Autodesk Inventor part; units mm, degrees
note: some values were not read from the file. Chosen so that the rebuilt part matches the saved one: direction of "Hole2".
(part 3 of 20)
  line L329 (-10082.582375, -10027.370137) -> (-10083.030705, -10031.210292)
  ellipse E243 centre (-10082.779407, -10029.059983) end of major axis (-10083.069525, -10031.543092) minor radius 0.000126 (-10083.029846, -10031.202932) -> (-10083.069521, -10031.543049) ccw
  line L330 (-10085.513815, -10030.920174) -> (-10085.181506, -10028.073798)
  ellipse E244 centre (-10085.262516, -10028.769865) end of major axis (-10085.552634, -10031.252974) minor radius 0.000126 (-10085.513815, -10030.920174) -> (-10085.552634, -10031.252974) ccw
  line L331 (-10083.069525, -10031.543092) -> (-10085.552634, -10031.252974)
  ellipse E245 centre (-10082.117991, -10023.398136) end of major axis (-10083.104393, -10031.840708) minor radius 0.000429 (-10083.054997, -10031.419086) -> (-10082.967028, -10030.666888) ccw
  line L332 (-10084.568877, -10027.13817) -> (-10084.684884, -10028.131821)
  ellipse E246 centre (-10082.643707, -10010.297398) end of major axis (-10082.614695, -10010.545709) minor radius 0.000013
  ellipse E247 centre (-10082.518842, -10011.365844) end of major axis (-10082.588111, -10010.772977) minor radius 0.00003 (-10082.582158, -10010.823819) -> (-10082.582182, -10010.823822) ccw
  ellipse E248 centre (-10082.117991, -10014.795845) end of major axis (-10083.104393, -10006.353274) minor radius 0.000429 (-10082.967028, -10007.527094) -> (-10083.054997, -10006.774896) ccw
  ellipse E249 centre (-10082.779407, -10009.133999) end of major axis (-10083.069525, -10006.650889) minor radius 0.000126 (-10083.054997, -10006.774896) -> (-10083.030705, -10006.983689) ccw
  line L333 (-10083.030705, -10006.983689) -> (-10082.582375, -10010.823844)
  line L334 (-10085.181506, -10010.120184) -> (-10085.513815, -10007.273807)
  ellipse E250 centre (-10085.262516, -10009.424117) end of major axis (-10085.552634, -10006.941007) minor radius 0.000126 (-10085.552634, -10006.941007) -> (-10085.513815, -10007.273807) ccw
  line L335 (-10085.552634, -10006.941007) -> (-10083.069525, -10006.650889)
  ellipse E251 centre (-10082.926301, -10007.876835) end of major axis (-10082.833946, -10008.667304) minor radius 0.000039 (-10082.96711, -10007.527248) -> (-10082.967167, -10007.527356) ccw
  line L336 (-10084.684884, -10010.06216) -> (-10084.568877, -10011.055811)
  line L337 (-10088.375684, -10026.030053) -> (-10088.470056, -10027.025887)
  line L338 (-10089.238176, -10029.831508) -> (-10088.967825, -10026.978705)
  ellipse E252 centre (-10089.033868, -10027.676195) end of major axis (-10089.269776, -10030.16504) minor radius 0.000028 (-10089.238176, -10029.831508) -> (-10089.269776, -10030.16504) ccw
  line L339 (-10087.361677, -10030.345901) -> (-10089.269776, -10030.16504)
  line L340 (-10088.55652, -10015.008914) -> (-10088.570909, -10015.096991)
  line L341 (-10088.570909, -10023.096991) -> (-10088.55652, -10023.185067)
  line L342 (-10088.777126, -10024.881551) -> (-10088.905304, -10024.096991)
  line L343 (-10088.905304, -10014.096991) -> (-10088.777126, -10013.312431)
  line L344 (-10088.470056, -10011.168095) -> (-10088.375684, -10012.163929)
  line L345 (-10088.967825, -10011.215277) -> (-10089.238176, -10008.362473)
  ellipse E253 centre (-10089.033868, -10010.517786) end of major axis (-10089.269776, -10008.028942) minor radius 0.000028 (-10089.269776, -10008.028942) -> (-10089.238179, -10008.362444) ccw
  line L346 (-10089.269776, -10008.028942) -> (-10087.361677, -10007.84808)
  spline S0 degree 3 poles (-10089.355394, -10025.372994) (-10089.375203, -10025.328104) (-10089.41441, -10025.239254) (-10089.470581, -10025.106444) (-10089.524077, -10024.975666) (-10089.590992, -10024.805344) (-10089.66863, -10024.596725) (-10089.723709, -10024.42915) (-10089.750761, -10024.346845) knots 0 0 0 0 0.13378969 0.26480564 0.39318317 0.51905417 0.76378306 1 1 1 1
  line L347 (-10088.828929, -10025.428076) -> (-10089.355394, -10025.372994)
  spline S1 degree 3 poles (-10089.713059, -10026.50077) (-10089.711978, -10026.51419) (-10089.709847, -10026.540646) (-10089.707768, -10026.579767) (-10089.706628, -10026.617583) (-10089.706543, -10026.653893) (-10089.707549, -10026.688508) (-10089.709676, -10026.721288) (-10089.712863, -10026.752152) (-10089.717058, -10026.781056) (-10089.722211, -10026.807959) (-10089.728269, -10026.832818) (-10089.735181, -10026.855595) (-10089.742902, -10026.876266) (-10089.751482, -10026.894991) (-10089.761038, -10026.911918) (-10089.771484, -10026.927357) (-10089.779493, -10026.936504) (-10089.783423, -10026.940992) knots 0 0 0 0 0.08847523 0.17442408 0.25743028 0.33708941 0.41301484 0.48496567 0.5529194 0.61687848 0.67685349 0.73286663 0.78495643 0.83318442 0.87777974 0.92016243 0.96082909 1 1 1 1
  ellipse E254 centre (-10089.027378, -10022.2409) end of major axis (-10089.595637, -10027.672254) minor radius 0.000387 (-10089.355394, -10025.372995) -> (-10089.595637, -10027.672254) ccw
  line L348 (-10089.849985, -10027.358464) -> (-10089.595637, -10027.672254)
  line L349 (-10089.039069, -10027.730485) -> (-10089.595637, -10027.672254)
  spline S2 degree 3 poles (-10089.491941, -10022.246911) (-10089.516181, -10022.204326) (-10089.564161, -10022.120035) (-10089.633469, -10021.993791) (-10089.69992, -10021.869289) (-10089.78374, -10021.706851) (-10089.882131, -10021.507435) (-10089.953949, -10021.346516) (-10089.989225, -10021.267475) knots 0 0 0 0 0.13376268 0.26475964 0.39312605 0.51899363 0.76373828 1 1 1 1
  line L350 (-10089.310215, -10022.246911) -> (-10089.491941, -10022.246911)
  line L351 (-10089.491941, -10015.94707) -> (-10089.310215, -10015.94707)
  spline S3 degree 3 poles (-10089.989225, -10016.926507) (-10089.953949, -10016.847466) (-10089.882131, -10016.686546) (-10089.78374, -10016.487131) (-10089.69992, -10016.324692) (-10089.633469, -10016.200191) (-10089.564161, -10016.073947) (-10089.516181, -10015.989656) (-10089.491941, -10015.94707) knots 0 0 0 0 0.23626172 0.48100637 0.60687395 0.73524036 0.86623732 1 1 1 1
  line L352 (-10089.989225, -10021.267475) -> (-10089.989225, -10016.926507)
  ellipse E255 centre (-10089.524961, -10019.096991) end of major axis (-10089.524961, -10024.057991) minor radius 0.5163 (-10089.959804, -10016.422408) -> (-10089.989225, -10016.926507) ccw
  ellipse E256 centre (-10089.524961, -10019.096991) end of major axis (-10089.524961, -10024.057991) minor radius 0.5163 (-10089.989225, -10021.267475) -> (-10089.959804, -10021.771573) ccw
  ellipse E257 centre (-10089.027676, -10019.096991) end of major axis (-10089.027676, -10013.635991) minor radius 0.568336 (-10089.165773, -10013.799655) -> (-10089.491941, -10015.94707) ccw
  ellipse E258 centre (-10089.027676, -10019.096991) end of major axis (-10089.027676, -10024.557991) minor radius 0.568336 (-10089.491941, -10022.246911) -> (-10089.165773, -10024.394327) ccw
  line L353 (-10089.355394, -10012.820988) -> (-10088.828929, -10012.765906)
  spline S4 degree 3 poles (-10089.750761, -10013.847136) (-10089.723709, -10013.764832) (-10089.66863, -10013.597256) (-10089.590992, -10013.388638) (-10089.524077, -10013.218316) (-10089.470581, -10013.087538) (-10089.41441, -10012.954727) (-10089.375203, -10012.865878) (-10089.355394, -10012.820988) knots 0 0 0 0 0.23621694 0.48094583 0.60681683 0.73519436 0.86621031 1 1 1 1
  spline S5 degree 3 poles (-10089.783618, -10011.253438) (-10089.779613, -10011.258107) (-10089.771405, -10011.267675) (-10089.76069, -10011.283901) (-10089.750805, -10011.301818) (-10089.74191, -10011.321545) (-10089.733975, -10011.343026) (-10089.727027, -10011.366257) (-10089.721076, -10011.391219) (-10089.716138, -10011.417899) (-10089.712225, -10011.446299) (-10089.709353, -10011.476466) (-10089.707507, -10011.508436) (-10089.70667, -10011.542209) (-10089.706829, -10011.57773) (-10089.707995, -10011.614936) (-10089.710092, -10011.653771) (-10089.712241, -10011.68016) (-10089.713337, -10011.693625) knots 0 0 0 0 0.04039145 0.08278851 0.12750015 0.17478558 0.22486002 0.27790108 0.33405492 0.39344169 0.45616024 0.52241148 0.59256068 0.66658365 0.74441779 0.82598879 0.91121312 1 1 1 1
  ellipse E259 centre (-10089.027378, -10015.953082) end of major axis (-10089.595637, -10010.521728) minor radius 0.000387 (-10089.595637, -10010.521728) -> (-10089.355394, -10012.820988) ccw
  line L354 (-10089.849985, -10010.835518) -> (-10089.595637, -10010.521728)
  line L355 (-10089.039069, -10010.463496) -> (-10089.595637, -10010.521728)
  spline S6 degree 3 poles (-10091.282091, -10024.900964) (-10091.302336, -10024.856269) (-10091.342408, -10024.767806) (-10091.39987, -10024.635549) (-10091.454637, -10024.505299) (-10091.523209, -10024.335637) (-10091.602875, -10024.127785) (-10091.659584, -10023.960754) (-10091.687437, -10023.878716) knots 0 0 0 0 0.13378969 0.26480564 0.39318317 0.51905417 0.76378306 1 1 1 1
  line L356 (-10089.484899, -10025.071313) -> (-10091.282091, -10024.900964)
  line L357 (-10091.687437, -10023.878716) -> (-10091.612013, -10023.082983)
  ellipse E260 centre (-10091.482604, -10021.718237) end of major axis (-10091.950739, -10026.6571) minor radius 0.000055 (-10091.93466, -10026.487305) -> (-10091.950739, -10026.6571) ccw
  ellipse E261 centre (-10091.482604, -10021.718237) end of major axis (-10091.950739, -10026.6571) minor radius 0.000055 (-10091.687437, -10023.878716) -> (-10091.814007, -10025.21415) ccw
  spline S7 degree 3 poles (-10091.814007, -10025.21415) (-10091.798163, -10025.265719) (-10091.767127, -10025.36673) (-10091.726257, -10025.516101) (-10091.691249, -10025.659093) (-10091.662778, -10025.794864) (-10091.640895, -10025.9237) (-10091.626418, -10026.045317) (-10091.620703, -10026.141851) (-10091.621057, -10026.213481) (-10091.623808, -10026.261718) (-10091.628873, -10026.305789) (-10091.636083, -10026.34554) (-10091.645286, -10026.380851) (-10091.659407, -10026.420321) (-10091.682241, -10026.461662) (-10091.720137, -10026.498843) (-10091.767469, -10026.519811) (-10091.821022, -10026.522371) (-10091.877958, -10026.511191) (-10091.915164, -10026.495517) (-10091.934659, -10026.487304) knots 0 0 0 0 0.10413454 0.20397599 0.29888876 0.38827472 0.47171081 0.55106733 0.62459732 0.65820388 0.68929134 0.71781594 0.74378428 0.76721832 0.78816557 0.82463321 0.85738378 0.88888098 0.92222056 0.95924484 1 1 1 1
  ellipse E262 centre (-10090.984835, -10021.765419) end of major axis (-10091.500152, -10027.202051) minor radius 0.000061 (-10091.282095, -10024.901006) -> (-10091.500152, -10027.202051) ccw
  line L358 (-10091.950739, -10026.6571) -> (-10091.500152, -10027.202051)
  ellipse E263 centre (-10091.808499, -10025.15622) end of major axis (-10091.665888, -10023.651664) minor radius 0.000017 (-10091.934703, -10026.487762) -> (-10091.821814, -10025.296875) ccw
  line L359 (-10089.849985, -10027.358464) -> (-10091.500152, -10027.202051)
  spline S8 degree 3 poles (-10091.405595, -10022.246911) (-10091.42986, -10022.204326) (-10091.477886, -10022.120036) (-10091.547262, -10021.993791) (-10091.613777, -10021.86929) (-10091.697679, -10021.706852) (-10091.796165, -10021.507438) (-10091.868055, -10021.346516) (-10091.903366, -10021.267475) knots 0 0 0 0 0.13376751 0.26476787 0.39313627 0.51900446 0.76374629 1 1 1 1
  line L360 (-10089.691497, -10022.246911) -> (-10091.405595, -10022.246911)
  line L361 (-10091.405595, -10015.94707) -> (-10089.691497, -10015.94707)
  spline S9 degree 3 poles (-10091.903366, -10016.926507) (-10091.868055, -10016.847466) (-10091.796165, -10016.686543) (-10091.697679, -10016.487129) (-10091.613777, -10016.324692) (-10091.547262, -10016.20019) (-10091.477886, -10016.073946) (-10091.42986, -10015.989656) (-10091.405595, -10015.94707) knots 0 0 0 0 0.23625371 0.48099554 0.60686373 0.73523213 0.86623249 1 1 1 1
  line L362 (-10091.903366, -10021.267475) -> (-10091.903366, -10016.926507)
  ellipse E264 centre (-10091.482582, -10019.096991) end of major axis (-10091.482582, -10024.057991) minor radius 0.467946 (-10091.813104, -10015.585157) -> (-10091.903366, -10016.926507) ccw
  ellipse E265 centre (-10091.482582, -10019.096991) end of major axis (-10091.482582, -10024.057991) minor radius 0.467946 (-10091.903366, -10021.267475) -> (-10091.813104, -10022.608825) ccw
  spline S10 degree 3 poles (-10091.813104, -10022.608825) (-10091.794916, -10022.648919) (-10091.759087, -10022.727902) (-10091.708202, -10022.845276) (-10091.6607, -10022.959182) (-10091.616959, -10023.069176) (-10091.577206, -10023.174758) (-10091.541408, -10023.276157) (-10091.509741, -10023.373699) (-10091.482497, -10023.466914) (-10091.460403, -10023.553917) (-10091.444493, -10023.632581) (-10091.434982, -10023.701386) (-10091.431489, -10023.75949) (-10091.433695, -10023.80769) (-10091.442096, -10023.846389) (-10091.455729, -10023.877879) (-10091.471318, -10023.891426) (-10091.478563, -10023.897722) knots 0 0 0 0 0.09648314 0.19006443 0.28034292 0.36693478 0.44946267 0.527566 0.60257164 0.67417927 0.74035842 0.79922956 0.84998037 0.89243012 0.92670891 0.95522625 0.97919149 1 1 1 1
  spline S11 degree 3 poles (-10091.478569, -10014.296272) (-10091.471499, -10014.302418) (-10091.456208, -10014.315713) (-10091.442744, -10014.346899) (-10091.434361, -10014.385571) (-10091.431755, -10014.433144) (-10091.434624, -10014.489116) (-10091.443205, -10014.553706) (-10091.457617, -10014.626897) (-10091.477678, -10014.708609) (-10091.503233, -10014.798357) (-10091.534062, -10014.895415) (-10091.569942, -10014.999051) (-10091.610624, -10015.108521) (-10091.655873, -10015.222921) (-10091.722241, -10015.383074) (-10091.776464, -10015.503669) (-10091.813104, -10015.585157) knots 0 0 0 0 0.02031374 0.04393674 0.07255557 0.10706143 0.14790384 0.19530387 0.24973648 0.31134419 0.37967367 0.4542385 0.53453299 0.62003981 0.71019877 0.8041769 1 1 1 1
  ellipse E266 centre (-10090.984812, -10019.096991) end of major axis (-10090.984812, -10013.635991) minor radius 0.515109 (-10091.154807, -10013.941946) -> (-10091.405595, -10015.94707) ccw
  ellipse E267 centre (-10090.984812, -10019.096991) end of major axis (-10090.984812, -10024.557991) minor radius 0.515109 (-10091.405595, -10022.246911) -> (-10091.154807, -10024.252035) ccw
  line L363 (-10091.282091, -10013.293017) -> (-10089.484899, -10013.122668)
  spline S12 degree 3 poles (-10091.687437, -10014.315265) (-10091.659584, -10014.233228) (-10091.602875, -10014.066197) (-10091.523209, -10013.858345) (-10091.454637, -10013.688683) (-10091.39987, -10013.558433) (-10091.342408, -10013.426176) (-10091.302336, -10013.337712) (-10091.282091, -10013.293017) knots 0 0 0 0 0.23621694 0.48094583 0.60681683 0.73519436 0.86621031 1 1 1 1
  line L364 (-10091.612013, -10015.110999) -> (-10091.687437, -10014.315265)
  ellipse E268 centre (-10091.482604, -10016.475744) end of major axis (-10091.014468, -10021.414608) minor radius 0.000055 (-10091.814145, -10012.978375) -> (-10091.687613, -10014.313411) ccw
  ellipse E269 centre (-10091.482604, -10016.475744) end of major axis (-10091.950739, -10011.536881) minor radius 0.000055 (-10091.950739, -10011.536881) -> (-10091.934659, -10011.706679) ccw
  spline S13 degree 3 poles (-10091.934659, -10011.706678) (-10091.914651, -10011.69823) (-10091.877086, -10011.68237) (-10091.820071, -10011.671463) (-10091.767544, -10011.674319) (-10091.721092, -10011.694698) (-10091.683481, -10011.731672) (-10091.654843, -10011.783177) (-10091.634672, -10011.848527) (-10091.622919, -10011.927815) (-10091.619845, -10012.021105) (-10091.624909, -10012.128035) (-10091.638005, -10012.247654) (-10091.658962, -10012.378555) (-10091.687598, -10012.519238) (-10091.723631, -10012.667871) (-10091.765738, -10012.822577) (-10091.79775, -10012.92687) (-10091.814007, -10012.979832) knots 0 0 0 0 0.04184874 0.07857029 0.11114659 0.14190435 0.17426777 0.21118388 0.25459927 0.30565856 0.36551927 0.43456112 0.51220716 0.59775966 0.69045627 0.7893544 0.8930296 1 1 1 1
  ellipse E270 centre (-10090.984835, -10016.428563) end of major axis (-10091.500152, -10010.991931) minor radius 0.000061 (-10091.500152, -10010.991931) -> (-10091.282091, -10013.293017) ccw
  line L365 (-10091.950739, -10011.536881) -> (-10091.500152, -10010.991931)
  line L366 (-10089.849985, -10010.835518) -> (-10091.500152, -10010.991931)
  ellipse E271 centre (-10092.011091, -10021.928727) end of major axis (-10092.418478, -10025.822473) minor radius 0.000278 (-10092.049003, -10022.288426) -> (-10092.181257, -10023.552725) ccw
  ellipse E272 centre (-10092.214166, -10023.867654) end of major axis (-10092.193354, -10023.66874) minor radius 0.000014 (-10092.202773, -10023.758879) -> (-10092.193354, -10023.66874) ccw
  line L367 (-10092.193376, -10023.668676) -> (-10092.193354, -10023.66874)
  ellipse E273 centre (-10092.172564, -10023.469762) end of major axis (-10092.193376, -10023.668676) minor radius 0.000014 (-10092.181257, -10023.552725) -> (-10092.193376, -10023.668676) ccw
  ellipse E274 centre (-10092.011091, -10021.928727) end of major axis (-10092.361246, -10025.275459) minor radius 0.000239 (-10092.202773, -10023.758879) -> (-10092.361246, -10025.275459) ccw
  line L368 (-10092.361246, -10025.275459) -> (-10091.825101, -10025.331553)
  ellipse E275 centre (-10107.725317, -10020.284613) end of major axis (-10107.960488, -10022.532344) minor radius 0.00016 (-10107.931882, -10022.258193) -> (-10107.960488, -10022.532344) ccw
  line L369 (-10107.960488, -10022.532344) -> (-10106.013379, -10022.828708)
  line L370 (-10091.903366, -10017.346991) -> (-10092.362753, -10017.346991)
  ellipse E276 centre (-10092.362753, -10017.546991) end of major axis (-10092.362753, -10017.346991) minor radius 0.020814 (-10092.362753, -10017.346991) -> (-10092.381669, -10017.463545) ccw
  ellipse E277 centre (-10092.011385, -10019.096991) end of major axis (-10092.011385, -10023.011991) minor radius 0.407441 (-10092.381669, -10017.463545) -> (-10092.381669, -10020.730436) ccw
  ellipse E278 centre (-10092.321979, -10017.146991) end of major axis (-10092.321979, -10017.346991) minor radius 0.020814 (-10092.321979, -10017.346991) -> (-10092.304554, -10017.256388) ccw
  ellipse E279 centre (-10092.321979, -10021.046991) end of major axis (-10092.321979, -10020.846991) minor radius 0.020814 (-10092.304554, -10020.937594) -> (-10092.321979, -10020.846991) ccw
  ellipse E280 centre (-10092.362753, -10020.646991) end of major axis (-10092.362753, -10020.846991) minor radius 0.020814 (-10092.381669, -10020.730436) -> (-10092.362753, -10020.846991) ccw
  line L371 (-10092.362753, -10020.846991) -> (-10091.903366, -10020.846991)
  ellipse E281 centre (-10092.011385, -10019.096991) end of major axis (-10092.011385, -10015.731991) minor radius 0.350202 (-10092.063275, -10015.769135) -> (-10092.304554, -10017.256388) ccw
  ellipse E282 centre (-10092.011385, -10019.096991) end of major axis (-10092.011385, -10022.461991) minor radius 0.350202 (-10092.304554, -10020.937594) -> (-10092.063275, -10022.424847) ccw
  ellipse E283 centre (-10107.725588, -10019.096991) end of major axis (-10107.725588, -10016.836991) minor radius 0.235202 (-10107.934511, -10018.058913) -> (-10107.934511, -10020.135069) ccw
  ellipse E284 centre (-10092.172564, -10014.724219) end of major axis (-10092.193376, -10014.525305) minor radius 0.000014 (-10092.193376, -10014.525305) -> (-10092.181257, -10014.641257) ccw
  ellipse E285 centre (-10092.011091, -10016.265255) end of major axis (-10091.603705, -10020.159001) minor radius 0.000278 (-10092.181259, -10014.641244) -> (-10092.049005, -10015.905542) ccw
  line L372 (-10092.193354, -10014.525241) -> (-10092.193376, -10014.525305)
  ellipse E286 centre (-10092.214166, -10014.326327) end of major axis (-10092.193354, -10014.525241) minor radius 0.000014 (-10092.193354, -10014.525241) -> (-10092.202773, -10014.435103) ccw
  ellipse E287 centre (-10092.011091, -10016.265255) end of major axis (-10092.361246, -10012.918523) minor radius 0.000239 (-10092.361246, -10012.918523) -> (-10092.202773, -10014.435105) ccw
  line L373 (-10092.361246, -10012.918523) -> (-10091.825101, -10012.862428)
  ellipse E288 centre (-10107.725317, -10017.909368) end of major axis (-10107.960488, -10015.661637) minor radius 0.00016 (-10107.960488, -10015.661637) -> (-10107.931882, -10015.935788) ccw
  line L374 (-10107.960488, -10015.661637) -> (-10106.013379, -10015.365274)
  ellipse E289 centre (-10105.757191, -10020.636212) end of major axis (-10106.019458, -10022.880943) minor radius 0.000114 (-10105.930965, -10022.122802) -> (-10106.019458, -10022.880943) ccw
  line L375 (-10106.019458, -10022.880943) -> (-10094.287038, -10024.811778)
  line L376 (-10093.990126, -10024.860641) -> (-10092.346221, -10025.131183)
  ellipse E290 centre (-10090.064389, -10019.096991) end of major axis (-10090.064389, -10023.011991) minor radius 0.45382 (-10090.510503, -10018.378625) -> (-10090.512583, -10018.482465) ccw
  ellipse E291 centre (-10090.064389, -10019.096991) end of major axis (-10090.064389, -10023.011991) minor radius 0.45382 (-10090.516487, -10018.756319) -> (-10090.515885, -10019.492622) ccw
  ellipse E292 centre (-10090.064389, -10019.096991) end of major axis (-10090.064389, -10023.011991) minor radius 0.45382 (-10090.512583, -10019.711517) -> (-10090.510503, -10019.815357) ccw
  ellipse E293 centre (-10105.757877, -10019.096991) end of major axis (-10105.757877, -10016.836991) minor radius 0.261975 (-10105.929305, -10017.38803) -> (-10105.929305, -10020.805951) ccw
  ellipse E294 centre (-10105.757191, -10017.55777) end of major axis (-10106.019458, -10015.313039) minor radius 0.000114 (-10106.019458, -10015.313039) -> (-10105.930965, -10016.07118) ccw
  line L377 (-10106.019458, -10015.313039) -> (-10094.287038, -10013.382204)
  line L378 (-10093.990126, -10013.33334) -> (-10092.346221, -10013.062799)
  ellipse E295 centre (-10110.685615, -10019.898058) end of major axis (-10110.66627, -10019.693973) minor radius 0.000002 (-10110.66627, -10019.693973) -> (-10110.689578, -10019.939846) ccw
  ellipse E296 centre (-10110.251606, -10019.939196) end of major axis (-10110.368144, -10021.168686) minor radius 0.000014 (-10110.284172, -10020.282632) -> (-10110.368144, -10021.168686) ccw
  line L379 (-10110.368144, -10021.168686) -> (-10109.817506, -10021.220878)
  arc A0 (-10110.696073, -10020.26555) -> (-10110.368144, -10021.168686) centre (-10108.775104, -10020.079148) ccw
  arc A1 (-10110.641595, -10019.588148) -> (-10110.66627, -10019.693973) centre (-10108.775104, -10020.079148) ccw
  ellipse E297 centre (-10093.971448, -10021.482329) end of major axis (-10094.34088, -10025.37986) minor radius 0.000044 (-10094.031971, -10022.120387) -> (-10094.125601, -10023.108231) ccw
  ellipse E298 centre (-10092.975911, -10021.576692) end of major axis (-10093.345342, -10025.474223) minor radius 0.000044 (-10092.99969, -10021.827109) -> (-10093.130063, -10023.202594) ccw
  line L380 (-10094.136599, -10023.224279) -> (-10094.136597, -10023.224307)
  line L381 (-10093.141061, -10023.318642) -> (-10093.141059, -10023.31867)
  ellipse E299 centre (-10093.971448, -10021.482329) end of major axis (-10094.28898, -10024.832314) minor radius 0.000037 (-10094.145146, -10023.314518) -> (-10094.28898, -10024.832314) ccw
  ellipse E300 centre (-10092.975911, -10021.576692) end of major axis (-10093.293443, -10024.926677) minor radius 0.000037 (-10093.149608, -10023.40888) -> (-10093.270588, -10024.685411) ccw
  line L382 (-10094.28898, -10024.832314) -> (-10093.990122, -10024.860642)
  ellipse E301 centre (-10109.700946, -10019.991391) end of major axis (-10109.914207, -10022.241307) minor radius 0.000025 (-10109.803801, -10021.076282) -> (-10109.914207, -10022.241307) ccw
  line L383 (-10109.914207, -10022.241307) -> (-10107.959153, -10022.519419)
  ellipse E302 centre (-10110.251653, -10019.096991) end of major axis (-10110.251653, -10017.861991) minor radius 0.116491 (-10110.284248, -10017.911323) -> (-10110.284248, -10020.282659) ccw
  arc A2 (-10110.694309, -10019.301148) -> (-10110.436834, -10020.078653) centre (-10108.775145, -10019.096991) ccw
  arc A3 (-10110.436834, -10018.115328) -> (-10110.694309, -10018.892833) centre (-10108.775145, -10019.096991) ccw
  ellipse E303 centre (-10093.294355, -10017.546991) end of major axis (-10093.294355, -10017.346991) minor radius 0.018865 (-10093.294355, -10017.346991) -> (-10093.311499, -10017.463545) ccw
  line L384 (-10093.294355, -10017.346991) -> (-10094.289896, -10017.346991)
  ellipse E304 centre (-10094.289896, -10017.546991) end of major axis (-10094.289896, -10017.346991) minor radius 0.018865 (-10094.289896, -10017.346991) -> (-10094.307041, -10017.463545) ccw
  ellipse E305 centre (-10093.971436, -10019.096991) end of major axis (-10093.971436, -10023.011991) minor radius 0.369282 (-10094.307041, -10017.463545) -> (-10094.307041, -10020.730436) ccw
  ellipse E306 centre (-10092.975894, -10019.096991) end of major axis (-10092.975894, -10023.011991) minor radius 0.369282 (-10093.311499, -10017.463545) -> (-10093.311499, -10020.730436) ccw
  ellipse E307 centre (-10094.252941, -10017.146991) end of major axis (-10094.252941, -10017.346991) minor radius 0.018865 (-10094.252941, -10017.346991) -> (-10094.237148, -10017.256388) ccw
  ellipse E308 centre (-10094.252941, -10021.046991) end of major axis (-10094.252941, -10020.846991) minor radius 0.018865 (-10094.237148, -10020.937594) -> (-10094.252941, -10020.846991) ccw
  ellipse E309 centre (-10094.289896, -10020.646991) end of major axis (-10094.289896, -10020.846991) minor radius 0.018865 (-10094.307041, -10020.730436) -> (-10094.289896, -10020.846991) ccw
  ellipse E310 centre (-10093.294355, -10020.646991) end of major axis (-10093.294355, -10020.846991) minor radius 0.018865 (-10093.311499, -10020.730436) -> (-10093.294355, -10020.846991) ccw
  line L385 (-10094.289896, -10020.846991) -> (-10093.294355, -10020.846991)
  ellipse E311 centre (-10093.257399, -10017.146991) end of major axis (-10093.257399, -10017.346991) minor radius 0.018865 (-10093.257399, -10017.346991) -> (-10093.241607, -10017.256388) ccw
  line L386 (-10093.257399, -10017.346991) -> (-10093.294355, -10017.346991)
  ellipse E312 centre (-10093.257399, -10021.046991) end of major axis (-10093.257399, -10020.846991) minor radius 0.018865 (-10093.241607, -10020.937594) -> (-10093.257399, -10020.846991) ccw
  line L387 (-10093.294355, -10020.846991) -> (-10093.257399, -10020.846991)
  ellipse E313 centre (-10093.971436, -10019.096991) end of major axis (-10093.971436, -10015.731991) minor radius 0.317404 (-10094.053503, -10015.846416) -> (-10094.237148, -10017.256388) ccw
  ellipse E314 centre (-10093.971436, -10019.096991) end of major axis (-10093.971436, -10022.461991) minor radius 0.317404 (-10094.237148, -10020.937594) -> (-10094.053503, -10022.347566) ccw
  ellipse E315 centre (-10092.975894, -10019.096991) end of major axis (-10092.975894, -10022.461991) minor radius 0.317404 (-10093.050842, -10022.366837) -> (-10093.015075, -10022.436255) ccw
  ellipse E316 centre (-10092.975894, -10019.096991) end of major axis (-10092.975894, -10015.731991) minor radius 0.317404 (-10093.241607, -10020.937594) -> (-10093.107762, -10022.157837) ccw
  ellipse E317 centre (-10092.975894, -10019.096991) end of major axis (-10092.975894, -10015.731991) minor radius 0.317404 (-10093.107762, -10016.036144) -> (-10093.241607, -10017.256388) ccw
  ellipse E318 centre (-10092.975894, -10019.096991) end of major axis (-10092.975894, -10015.731991) minor radius 0.317404 (-10093.015075, -10015.757727) -> (-10093.050842, -10015.827145) ccw
  ellipse E319 centre (-10109.700991, -10019.096991) end of major axis (-10109.700991, -10016.836991) minor radius 0.213175 (-10109.803832, -10017.117374) -> (-10109.803832, -10021.076608) ccw
  ellipse E320 centre (-10110.685615, -10018.295923) end of major axis (-10110.66627, -10018.500009) minor radius 0.000002 (-10110.689578, -10018.254136) -> (-10110.66627, -10018.500009) ccw
  ellipse E321 centre (-10110.251606, -10018.254785) end of major axis (-10110.368144, -10017.025296) minor radius 0.000014 (-10110.368144, -10017.025296) -> (-10110.284172, -10017.91135) ccw
  line L388 (-10110.368144, -10017.025296) -> (-10109.817506, -10016.973103)
  arc A4 (-10110.66627, -10018.500009) -> (-10110.641595, -10018.605833) centre (-10108.775104, -10018.114833) ccw
  arc A5 (-10110.368144, -10017.025296) -> (-10110.696073, -10017.928432) centre (-10108.775104, -10018.114833) ccw
  ellipse E322 centre (-10093.971448, -10016.711652) end of major axis (-10093.602017, -10020.609183) minor radius 0.000044 (-10094.12565, -10015.085235) -> (-10094.032024, -10016.073035) ccw
  ellipse E323 centre (-10092.975911, -10016.617289) end of major axis (-10092.606479, -10020.51482) minor radius 0.000044 (-10093.130112, -10014.990873) -> (-10092.999744, -10016.366308) ccw
  line L389 (-10094.136597, -10014.969675) -> (-10094.136599, -10014.969703)
  line L390 (-10093.141059, -10014.875312) -> (-10093.141061, -10014.87534)
  ellipse E324 centre (-10093.971448, -10016.711652) end of major axis (-10094.28898, -10013.361668) minor radius 0.000037 (-10094.28898, -10013.361668) -> (-10094.145137, -10014.879558) ccw
  ellipse E325 centre (-10092.975911, -10016.617289) end of major axis (-10093.293443, -10013.267304) minor radius 0.000037 (-10093.270588, -10013.50857) -> (-10093.149608, -10014.7851) ccw
  line L391 (-10094.28898, -10013.361668) -> (-10093.990122, -10013.33334)
  ellipse E326 centre (-10109.700946, -10018.20259) end of major axis (-10109.914207, -10015.952675) minor radius 0.000025 (-10109.914207, -10015.952675) -> (-10109.803801, -10017.117699) ccw
  line L392 (-10109.914207, -10015.952675) -> (-10107.959153, -10015.674562)
  line L393 (-10057.500001, -10011.931756) -> (-10059.215205, -10012.597408)
  line L394 (-10057.500001, -10009.857036) -> (-10059.380605, -10010.399295)
  line L395 (-10057.500001, -10028.891036) -> (-10059.519229, -10028.993122)
  line L396 (-10057.500001, -10026.820751) -> (-10059.450944, -10026.718216)
  line L397 (-10058.162515, -10011.976262) -> (-10059.262653, -10012.20944)
  line L398 (-10058.216133, -10009.845213) -> (-10059.471021, -10009.986737)
  line L399 (-10058.216133, -10028.348769) -> (-10059.471021, -10028.207244)
  line L400 (-10058.162515, -10026.217719) -> (-10059.262653, -10025.984541)
  line L401 (-10057.500001, -10011.373231) -> (-10059.450944, -10011.475766)
  line L402 (-10057.500001, -10009.302945) -> (-10059.500161, -10009.201823)
  line L403 (-10057.500001, -10028.336946) -> (-10059.388385, -10027.792443)
  line L404 (-10057.500001, -10026.262225) -> (-10059.215205, -10025.596574)
  line L405 (-10058.910713, -10011.69724) -> (-10059.356318, -10011.779934)
  line L406 (-10058.896142, -10009.511335) -> (-10059.517424, -10009.572028)
  line L407 (-10058.896142, -10028.682647) -> (-10059.517424, -10028.621954)
  line L408 (-10058.910713, -10026.496741) -> (-10059.356318, -10026.414048)
  ellipse E327 centre (-10072.750524, -10029.519932) end of major axis (-10072.925788, -10029.593298) minor radius 0.172083 (-10072.758689, -10029.694739) -> (-10072.583874, -10029.588813) ccw
  ellipse E328 centre (-10072.72597, -10029.578588) end of major axis (-10072.550706, -10029.505222) minor radius 0.172083 (-10072.617768, -10029.713907) -> (-10072.56398, -10029.65569) ccw
  ellipse E329 centre (-10069.946648, -10029.508558) end of major axis (-10070.121912, -10029.581924) minor radius 0.172083 (-10070.098511, -10029.620791) -> (-10070.078788, -10029.640963) ccw
  ellipse E330 centre (-10072.72763, -10029.769957) end of major axis (-10072.537837, -10029.778821) minor radius 0.073999 (-10072.540371, -10029.765239) -> (-10072.758732, -10029.695659) ccw
  ellipse E331 centre (-10072.734076, -10029.907963) end of major axis (-10072.544283, -10029.916827) minor radius 0.073999 (-10072.546816, -10029.903244) -> (-10072.765177, -10029.833665) ccw
  ellipse E332 centre (-10069.954754, -10029.837932) end of major axis (-10070.144547, -10029.829068) minor radius 0.073999 (-10069.985855, -10029.763634) -> (-10070.142013, -10029.842651) ccw
  ellipse E333 centre (-10069.971202, -10029.449901) end of major axis (-10070.146466, -10029.523267) minor radius 0.172083 (-10070.129253, -10029.554068) -> (-10069.979366, -10029.624709) ccw
  ellipse E334 centre (-10069.948308, -10029.699927) end of major axis (-10070.138101, -10029.691062) minor radius 0.073999 (-10069.979409, -10029.625629) -> (-10070.138101, -10029.691062) ccw
  line L409 (-10070.138101, -10029.691062) -> (-10070.144547, -10029.829068)
  line L410 (-10072.531336, -10029.415958) -> (-10072.535588, -10029.507006)
  line L411 (-10072.559434, -10029.433185) -> (-10072.553878, -10029.314245)
  line L412 (-10070.288981, -10028.828886) -> (-10070.723556, -10028.839836)
  line L413 (-10072.122572, -10028.875087) -> (-10072.319266, -10028.880043)
  line L414 (-10072.447321, -10030.140928) -> (-10072.546816, -10029.903244)
  line L415 (-10072.540371, -10029.765239) -> (-10072.485677, -10029.895898)
  line L416 (-10070.142013, -10029.842651) -> (-10070.099909, -10029.943233)
  line L417 (-10070.196682, -10030.164113) -> (-10072.226967, -10030.21527)
  line L418 (-10070.148764, -10029.247005) -> (-10070.152568, -10029.32844)
  line L419 (-10072.220521, -10030.077265) -> (-10070.190236, -10030.026108)
  line L420 (-10072.34382, -10028.821387) -> (-10072.10911, -10028.815473)
  line L421 (-10071.080922, -10028.789566) -> (-10070.313535, -10028.77023)
  ellipse E335 centre (-10074.105776, -10029.613355) end of major axis (-10074.281039, -10029.686721) minor radius 0.172083 (-10074.281039, -10029.686721) -> (-10074.237915, -10029.74576) ccw
  ellipse E336 centre (-10068.566843, -10029.473791) end of major axis (-10068.391579, -10029.400425) minor radius 0.172083 (-10068.45864, -10029.60911) -> (-10068.443895, -10029.59737) ccw
  ellipse E337 centre (-10068.591397, -10029.415135) end of major axis (-10068.76666, -10029.488501) minor radius 0.172083 (-10068.599561, -10029.589942) -> (-10068.459535, -10029.530433) ccw
  ellipse E338 centre (-10074.130329, -10029.554699) end of major axis (-10074.305593, -10029.628065) minor radius 0.172083 (-10074.31093, -10029.61326) -> (-10074.138494, -10029.729506) ccw
  line L422 (-10074.281039, -10029.686721) -> (-10074.305593, -10029.628065)
  line L423 (-10068.37857, -10029.447377) -> (-10068.331245, -10028.434115)
  line L424 (-10068.599561, -10029.589942) -> (-10069.979366, -10029.624709)
  line L425 (-10068.386031, -10029.022741) -> (-10068.402416, -10029.373556)
  line L426 (-10074.307602, -10029.345598) -> (-10074.305333, -10029.297026)
  line L427 (-10072.758689, -10029.694739) -> (-10074.138494, -10029.729506)
  ellipse E339 centre (-10070.297146, -10029.003694) end of major axis (-10070.121882, -10028.930328) minor radius 0.172083 (-10070.174524, -10028.863699) -> (-10070.288981, -10028.828886) ccw
  ellipse E340 centre (-10072.327431, -10029.05485) end of major axis (-10072.152167, -10028.981484) minor radius 0.172083 (-10072.319266, -10028.880043) -> (-10072.37099, -10028.888055) ccw
  ellipse E341 centre (-10070.227783, -10030.089815) end of major axis (-10070.03799, -10030.09868) minor radius 0.073999 (-10070.196682, -10030.164113) -> (-10070.094884, -10030.147965) ccw
  ellipse E342 centre (-10072.258068, -10030.140972) end of major axis (-10072.447861, -10030.132108) minor radius 0.073999 (-10072.437026, -10030.158584) -> (-10072.226967, -10030.21527) ccw
  ellipse E343 centre (-10072.351984, -10028.996194) end of major axis (-10072.527248, -10029.06956) minor radius 0.172083 (-10072.34382, -10028.821387) -> (-10072.442566, -10028.849438) ccw
  ellipse E344 centre (-10070.3217, -10028.945037) end of major axis (-10070.146436, -10028.871671) minor radius 0.172083 (-10070.172307, -10028.829862) -> (-10070.313535, -10028.77023) ccw
  ellipse E345 centre (-10070.221338, -10029.95181) end of major axis (-10070.411131, -10029.942945) minor radius 0.073999 (-10070.190236, -10030.026108) -> (-10070.109169, -10030.016005) ccw
  ellipse E346 centre (-10072.251623, -10030.002967) end of major axis (-10072.441416, -10029.994102) minor radius 0.073999 (-10072.293271, -10030.073579) -> (-10072.220521, -10030.077265) ccw
  line L428 (-10072.765177, -10029.833665) -> (-10074.144982, -10029.868431)
  line L429 (-10074.30114, -10029.947448) -> (-10074.223731, -10030.13237)
  line L430 (-10068.200631, -10030.24531) -> (-10068.387689, -10029.798447)
  line L431 (-10068.60605, -10029.728867) -> (-10069.985855, -10029.763634)
  line L432 (-10072.758732, -10029.695659) -> (-10074.138537, -10029.730426)
  line L433 (-10068.599604, -10029.590862) -> (-10069.979409, -10029.625629)
  line L434 (-10068.024396, -10030.512914) -> (-10068.381243, -10029.660441)
  ellipse E347 centre (-10074.113881, -10029.942729) end of major axis (-10074.303674, -10029.933865) minor radius 0.073999 (-10074.144982, -10029.868431) -> (-10074.30114, -10029.947448) ccw
  ellipse E348 centre (-10068.574948, -10029.803165) end of major axis (-10068.385155, -10029.81203) minor radius 0.073999 (-10068.387689, -10029.798447) -> (-10068.60605, -10029.728867) ccw
  ellipse E349 centre (-10074.107435, -10029.804724) end of major axis (-10074.297229, -10029.795859) minor radius 0.073999 (-10074.138537, -10029.730426) -> (-10074.297229, -10029.795859) ccw
  ellipse E350 centre (-10068.568503, -10029.66516) end of major axis (-10068.37871, -10029.674024) minor radius 0.073999 (-10068.381243, -10029.660441) -> (-10068.599604, -10029.590862) ccw
  line L435 (-10074.303674, -10029.933865) -> (-10074.297229, -10029.795859)
  line L436 (-10067.943013, -10029.744417) -> (-10067.97273, -10030.380665)
  line L437 (-10067.948176, -10030.439322) -> (-10067.915655, -10029.743034)
  ellipse E351 centre (-10068.013653, -10030.282905) end of major axis (-10068.007356, -10030.532826) minor radius 0.041852 (-10068.024396, -10030.512914) -> (-10067.97273, -10030.380665) ccw
  ellipse E352 centre (-10068.013653, -10030.282905) end of major axis (-10068.003577, -10030.682778) minor radius 0.066962 (-10068.010366, -10030.680917) -> (-10067.948176, -10030.439322) ccw
  line L438 (-10068.009488, -10030.682927) -> (-10068.003577, -10030.682778)
  line L439 (-10072.587508, -10009.655971) -> (-10072.597938, -10009.375051)
  line L440 (-10070.348002, -10009.523828) -> (-10071.617541, -10009.65677)
  ellipse E353 centre (-10074.179771, -10009.488655) end of major axis (-10074.368132, -10009.513559) minor radius 0.101721 (-10074.275162, -10009.409276) -> (-10074.368565, -10009.508425) ccw
  line L441 (-10074.368565, -10009.508425) -> (-10074.364732, -10009.611686)
  line L442 (-10068.38674, -10009.420235) -> (-10068.397683, -10009.125503)
  line L443 (-10068.39807, -10009.115064) -> (-10068.400615, -10009.046522)
  line L444 (-10068.367861, -10009.607062) -> (-10068.371807, -10009.500763)
  ellipse E354 centre (-10070.351788, -10009.421853) end of major axis (-10070.163427, -10009.396949) minor radius 0.101721 (-10070.348002, -10009.523828) -> (-10070.170901, -10009.434254) ccw
  ellipse E355 centre (-10072.398714, -10009.636201) end of major axis (-10072.587075, -10009.661105) minor radius 0.101721 (-10072.587508, -10009.655971) -> (-10072.587494, -10009.656324) ccw
  line L445 (-10074.348285, -10028.471232) -> (-10074.348428, -10028.561211)
  line L446 (-10068.385905, -10028.805934) -> (-10068.385843, -10028.766317)
  line L447 (-10068.385543, -10028.577337) -> (-10068.385177, -10028.34651)
  line L448 (-10068.573855, -10028.253615) -> (-10069.267165, -10028.181013)
  line L449 (-10068.369056, -10028.682685) -> (-10068.368946, -10028.613538)
  ellipse E356 centre (-10068.573971, -10028.32674) end of major axis (-10068.385384, -10028.349871) minor radius 0.072673 (-10068.385177, -10028.34651) -> (-10068.573855, -10028.253615) ccw
  line L450 (-10070.154124, -10028.315431) -> (-10070.154194, -10028.35911)
  ellipse E357 centre (-10074.303434, -10028.194376) end of major axis (-10074.345093, -10028.592201) minor radius 0.017093 (-10074.348428, -10028.561211) -> (-10074.345093, -10028.592201) ccw
  line L451 (-10074.345093, -10028.592201) -> (-10074.340193, -10028.592714)
  line L452 (-10068.025544, -10007.68326) -> (-10067.992867, -10008.072468)
  line L453 (-10067.931233, -10008.45016) -> (-10068.002463, -10007.601765)
  ellipse E358 centre (-10068.212803, -10007.678541) end of major axis (-10068.029994, -10007.730317) minor radius 0.156811 (-10068.025544, -10007.68326) -> (-10068.06048, -10007.598817) ccw
  ellipse E359 centre (-10068.189722, -10007.597047) end of major axis (-10068.006913, -10007.648823) minor radius 0.156811 (-10068.002463, -10007.601765) -> (-10068.039279, -10007.514994) ccw
  line L454 (-10074.295747, -10008.422882) -> (-10074.304623, -10008.454219)
  line L455 (-10068.391172, -10008.60322) -> (-10068.266622, -10008.163465)
  line L456 (-10068.347095, -10008.610786) -> (-10068.045156, -10007.544709)
  line L457 (-10072.550299, -10008.498422) -> (-10072.461052, -10008.18331)
  line L458 (-10072.244556, -10008.084802) -> (-10070.214271, -10008.135959)
  ellipse E360 centre (-10072.522117, -10008.834092) end of major axis (-10072.512041, -10008.434219) minor radius 0.066962 (-10072.550299, -10008.498422) -> (-10072.583766, -10008.723327) ccw
  line L459 (-10072.549648, -10009.4566) -> (-10072.578231, -10009.116154)
  ellipse E361 centre (-10072.522117, -10008.834092) end of major axis (-10072.528414, -10009.084013) minor radius 0.041852 (-10072.564285, -10008.849906) -> (-10072.561065, -10008.963974) ccw
  line L460 (-10072.495409, -10008.467808) -> (-10072.513936, -10008.533223)
  ellipse E362 centre (-10070.117313, -10008.894685) end of major axis (-10070.127389, -10009.294559) minor radius 0.066962 (-10070.148166, -10008.568865) -> (-10070.182533, -10008.844399) ccw
  line L461 (-10072.324712, -10009.553664) -> (-10072.071304, -10009.560049)
  ellipse E363 centre (-10072.273792, -10008.188029) end of major axis (-10072.463126, -10008.203925) minor radius 0.102463 (-10072.244556, -10008.084802) -> (-10072.461052, -10008.18331) ccw
  ellipse E364 centre (-10070.243507, -10008.239186) end of major axis (-10070.432841, -10008.255082) minor radius 0.102463 (-10070.099438, -10008.163884) -> (-10070.214271, -10008.135959) ccw
  ellipse E365 centre (-10072.338098, -10009.394221) end of major axis (-10072.520908, -10009.342445) minor radius 0.156811 (-10072.389418, -10009.542483) -> (-10072.324712, -10009.553664) ccw
  ellipse E366 centre (-10072.36118, -10009.475716) end of major axis (-10072.17837, -10009.527492) minor radius 0.156811 (-10072.53924, -10009.510764) -> (-10072.44977, -10009.60805) ccw
  line L462 (-10068.343763, -10009.761902) -> (-10068.368688, -10009.465029)
  line L463 (-10068.39656, -10009.133047) -> (-10068.401458, -10009.074713)
  ellipse E367 centre (-10068.362989, -10008.938889) end of major axis (-10068.356692, -10008.688968) minor radius 0.041852 (-10068.404602, -10008.929751) -> (-10068.401458, -10009.074713) ccw
  ellipse E368 centre (-10074.276441, -10008.789888) end of major axis (-10074.286516, -10009.189761) minor radius 0.066962 (-10074.304623, -10008.454219) -> (-10074.34242, -10008.757756) ccw
  ellipse E369 centre (-10068.362989, -10008.938889) end of major axis (-10068.373065, -10009.338762) minor radius 0.066962 (-10068.391172, -10008.60322) -> (-10068.419347, -10008.767855) ccw
  ellipse E370 centre (-10068.232415, -10007.539991) end of major axis (-10068.043081, -10007.524095) minor radius 0.102463 (-10068.045156, -10007.544709) -> (-10068.042979, -10007.525546) ccw
  line L464 (-10067.987937, -10010.029885) -> (-10068.000487, -10010.074195)
  ellipse E371 centre (-10072.71748, -10029.857933) end of major axis (-10072.891596, -10029.933984) minor radius 0.168992 (-10072.723308, -10030.030204) -> (-10072.561349, -10029.939916) ccw
  ellipse E372 centre (-10072.690037, -10029.920762) end of major axis (-10072.515921, -10029.844712) minor radius 0.168992 (-10072.577401, -10030.048958) -> (-10072.53107, -10029.998422) ccw
  ellipse E373 centre (-10072.688578, -10030.110695) end of major axis (-10072.498687, -10030.117119) minor radius 0.079929 (-10072.501876, -10030.101256) -> (-10072.723339, -10030.031111) ccw
  ellipse E374 centre (-10072.69318, -10030.246698) end of major axis (-10072.503288, -10030.253123) minor radius 0.079929 (-10072.506477, -10030.237259) -> (-10072.72794, -10030.167115) ccw
  ellipse E375 centre (-10069.922125, -10030.106602) end of major axis (-10070.112017, -10030.100178) minor radius 0.079929 (-10069.956886, -10030.027019) -> (-10070.108828, -10030.116042) ccw
  ellipse E376 centre (-10069.946425, -10029.717837) end of major axis (-10070.120541, -10029.793888) minor radius 0.168992 (-10070.070615, -10029.856083) -> (-10069.952254, -10029.890109) ccw
  ellipse E377 centre (-10069.917524, -10029.970599) end of major axis (-10070.107415, -10029.964174) minor radius 0.079929 (-10069.952284, -10029.891015) -> (-10070.107415, -10029.964174) ccw
  line L465 (-10070.107415, -10029.964174) -> (-10070.112017, -10030.100178)
  line L466 (-10072.498932, -10029.78119) -> (-10072.501531, -10029.858022)
  line L467 (-10072.528889, -10029.792668) -> (-10072.526341, -10029.717381)
  line L468 (-10070.269411, -10029.120434) -> (-10070.627077, -10029.138516)
  line L469 (-10072.101739, -10029.21307) -> (-10072.293656, -10029.222773)
  line L470 (-10072.393048, -10030.496953) -> (-10072.506477, -10030.237259)
  line L471 (-10072.501876, -10030.101256) -> (-10072.388447, -10030.360949)
  line L472 (-10072.107645, -10031.150376) -> (-10072.213756, -10030.907437)
  line L473 (-10072.061815, -10030.818414) -> (-10070.037569, -10030.716075)
  line L474 (-10069.816107, -10030.786219) -> (-10069.709995, -10031.029159)
  line L475 (-10070.108828, -10030.116042) -> (-10069.995398, -10030.375735)
  line L476 (-10070.14734, -10030.464758) -> (-10072.171585, -10030.567098)
  line L477 (-10070.130246, -10029.642119) -> (-10070.13129, -10029.672972)
  line L478 (-10072.166984, -10030.431094) -> (-10070.142738, -10030.328755)
  ellipse E378 centre (-10072.095375, -10030.7877) end of major axis (-10072.075178, -10031.18719) minor radius 0.071491 (-10072.107645, -10031.150376) -> (-10072.022194, -10030.955245) ccw
  line L479 (-10072.017489, -10030.816173) -> (-10072.022194, -10030.955245)
  line L480 (-10072.049637, -10030.892415) -> (-10072.047686, -10030.834765)
  ellipse E379 centre (-10072.095375, -10030.7877) end of major axis (-10072.082751, -10031.037381) minor radius 0.044682 (-10072.103044, -10031.014373) -> (-10072.049637, -10030.892415) ccw
  line L481 (-10072.177108, -10030.844805) -> (-10072.103044, -10031.014373)
  ellipse E380 centre (-10069.697725, -10030.666483) end of major axis (-10069.677528, -10031.065972) minor radius 0.071491 (-10069.709995, -10031.029159) -> (-10069.677528, -10031.065972) ccw
  line L482 (-10072.321099, -10029.159944) -> (-10072.037847, -10029.145624)
  line L483 (-10070.647487, -10029.075331) -> (-10070.296853, -10029.057605)
  ellipse E381 centre (-10074.065738, -10029.990313) end of major axis (-10074.239854, -10030.066364) minor radius 0.168992 (-10074.239854, -10030.066364) -> (-10074.199948, -10030.120511) ccw
  ellipse E382 centre (-10068.543282, -10029.711116) end of major axis (-10068.369166, -10029.635065) minor radius 0.168992 (-10068.357771, -10029.716514) -> (-10068.35658, -10029.701676) ccw
  ellipse E383 centre (-10068.570725, -10029.648286) end of major axis (-10068.74484, -10029.724337) minor radius 0.168992 (-10068.385157, -10029.653236) -> (-10068.384022, -10029.638847) ccw
  ellipse E384 centre (-10068.570725, -10029.648286) end of major axis (-10068.74484, -10029.724337) minor radius 0.168992 (-10068.576553, -10029.820558) -> (-10068.503514, -10029.803338) ccw
  ellipse E385 centre (-10074.09318, -10029.927484) end of major axis (-10074.267296, -10030.003535) minor radius 0.168992 (-10074.269809, -10029.99742) -> (-10074.099009, -10030.099756) ccw
  line L484 (-10074.239854, -10030.066364) -> (-10074.267296, -10030.003535)
  line L485 (-10068.35658, -10029.701676) -> (-10068.356017, -10029.685043)
  line L486 (-10068.350877, -10029.53311) -> (-10068.313877, -10028.439522)
  line L487 (-10068.576553, -10029.820558) -> (-10069.952254, -10029.890109)
  line L488 (-10068.374848, -10029.367682) -> (-10068.377642, -10029.450251)
  line L489 (-10068.38333, -10029.618378) -> (-10068.384022, -10029.638847)
  line L490 (-10074.273984, -10029.762591) -> (-10074.27338, -10029.744731)
  line L491 (-10072.723308, -10030.030204) -> (-10074.099009, -10030.099756)
  ellipse E386 centre (-10070.275239, -10029.292705) end of major axis (-10070.101123, -10029.216654) minor radius 0.168992 (-10070.188964, -10029.133405) -> (-10070.269411, -10029.120434) ccw
  ellipse E387 centre (-10072.299485, -10029.395044) end of major axis (-10072.125369, -10029.318994) minor radius 0.168992 (-10072.293656, -10029.222773) -> (-10072.338893, -10029.230145) ccw
  ellipse E388 centre (-10072.027054, -10030.897998) end of major axis (-10072.216945, -10030.891573) minor radius 0.079929 (-10072.061815, -10030.818414) -> (-10072.213756, -10030.907437) ccw
  ellipse E389 centre (-10070.002809, -10030.795658) end of major axis (-10069.812917, -10030.802083) minor radius 0.079929 (-10069.816107, -10030.786219) -> (-10070.037569, -10030.716075) ccw
  ellipse E390 centre (-10070.1821, -10030.385175) end of major axis (-10069.992209, -10030.391599) minor radius 0.079929 (-10070.14734, -10030.464758) -> (-10069.995398, -10030.375735) ccw
  ellipse E391 centre (-10072.206346, -10030.487514) end of major axis (-10072.396237, -10030.481089) minor radius 0.079929 (-10072.393048, -10030.496953) -> (-10072.171585, -10030.567098) ccw